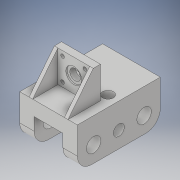
# Autodesk Inventor part: Y_Slider_Part_mit_Schrittmotor
Saved by Autodesk Inventor 2019 (Build 230136000, 136)
## iProperties
Created: 2018-08-19
Part Number: Y_Slider_Part_mit_Schrittmotor
Material: Generic
Document SubType Name: Modeling
Designer: Julia
Density: 1 g/cm^3
Appearance: Default
Author: Julia
Autodesk Inventor part; units mm, degrees
ref_plane "YZ Plane" through (0, 0, 0) normal (1, 0, 0) x (0, 1, 0)
ref_plane "XZ Plane" through (0, 0, 0) normal (0, 1, 0) x (-1, 0, 0)
ref_plane "XY Plane" through (0, 0, 0) normal (0, 0, 1) x (1, 0, 0)
sketch "Sketch1" plane through (0, 0, 0) normal (0, 1, 0) x (-1, 0, 0)
  line L0 (40, 57.5) -> (-40, 57.5)
  line L1 (-40, 57.5) -> (-40, -57.5)
  line L2 (-40, -57.5) -> (40, -57.5)
  line L3 (40, -57.5) -> (40, 57.5)
  point P0 (0, 0)
  point P1 (40, 0)
  point P2 (0, 57.5)
  dimension "d0" = 115
  dimension "d1" = 80
  constraints: 8 end point, 2 midpoint, 2 parallel, 1 horizontal, 1 horizontal alignment, 1 perpendicular, 1 vertical alignment
  measures "d0" distance of L2.end L0.start
  measures "d1" distance of L1.end L2.end
extrude "Extrusion1" add sketch "Sketch1" along normal blind 20
sketch "Sketch12" plane through (0, 0, 0) normal (0, -1, 0) x (1, 0, 0)
  line L0 (-40, 57.5) -> (-20, 57.5)
  line L1 (-20, 57.5) -> (-20, -57.5)
  line L2 (-20, -57.5) -> (-40, -57.5)
  line L3 (-40, -57.5) -> (-40, 57.5)
  line L4 (-40, -57.5) -> (-40, 57.5) projected
  line L5 (0, 100.8809) -> (0, -116.5773) construction
  line L6 (40, 57.5) -> (20, 57.5)
  line L7 (20, 57.5) -> (20, -57.5)
  line L8 (20, -57.5) -> (40, -57.5)
  line L9 (40, -57.5) -> (40, 57.5)
  point P0 (0, 0)
  point P1 (-40, 0)
  point P2 (0, 0)
  point P3 (-20, 0)
  dimension "d56" = 20
  dimension "d57" = 115
  constraints: 18 end point, 4 symmetric about line, 2 horizontal alignment, 2 midpoint, 2 parallel, 2 vertical, 1 collinear, 1 horizontal, 1 perpendicular
  measures "d56" distance of L0.start L0.end
  measures "d57" distance between parallel lines of L2 L0
extrude "Extrusion11" add sketch "Sketch12" along normal blind 37.5
sketch "Sketch13" plane through (-40, 0, 57.5) normal (-1, 0, 0) x (0, 0, 1)
  line L0 (0, 0) -> (-115, 0) projected
  point P0 (-57.5, 0)
  point P1 (-22.5, -15)
  point P2 (-92.5, -15)
  point P3 (-57.5, -15)
  point P4 (-57.5, 0)
  dimension "d129" = 35
  dimension "d130" = 35
  dimension "d131" = 15
  constraints: 2 horizontal alignment, 1 midpoint, 1 vertical alignment
  measures "d129" horizontal distance of point (-57.5, 0) point (-92.5, -15)
  measures "d130" horizontal distance of point (-22.5, -15) point (-57.5, 0)
  measures "d131" distance of point (-57.5, 0) point (-57.5, -15)
hole "Hole2" at (-40, -15, 35) at (-40, -15, -35) direction (1, 0, 0) diameter 20 end through all
hole "Hole3" at (-40, -15, 0) direction (1, 0, 0) diameter 15 end through all
sketch "Sketch19" plane through (0, 20, 0) normal (0, 1, 0) x (1, 0, 0)
  point P0 (0, 0)
  point P1 (25, 0)
  point P2 (-25, 0)
  dimension "d111" = 25
  dimension "d112" = 25
  constraints: 2 horizontal alignment
  measures "d111" distance of point (0, 0) point (25, 0)
  measures "d112" distance of point (-25, 0) point (0, 0)
hole "Hole6" at (25, 20, 0) at (-25, 20, 0) direction (0, -1, 0) diameter 15 depth 15
fillet "Fillet19" radius 20 4 edges at (-30, -37.5, -57.5) (30, -37.5, -57.5) (30, -37.5, 57.5) (-30, -37.5, 57.5)
sketch "Sketch20" plane through (0, 20, 0) normal (0, 1, 0) x (1, 0, 0)
  line L0 (-27, -22.5) -> (27, -22.5)
  line L1 (27, -22.5) -> (27, -12.5)
  line L2 (27, -12.5) -> (-27, -12.5)
  line L3 (-27, -12.5) -> (-27, -22.5)
  line L4 (-40, 57.5) -> (-40, -57.5) projected
  line L5 (40, -57.5) -> (40, 57.5) projected
  line L6 (-40, -57.5) -> (40, -57.5) projected
  point P0 (0, 0)
  point P1 (0, -12.5)
  dimension "d122" = 10
  dimension "d151" = 45
  dimension "d152" = 54
  constraints: 8 end point, 2 parallel, 1 horizontal, 1 midpoint, 1 perpendicular, 1 vertical alignment
  measures "d122" distance between parallel lines of L0 L2
  measures "d151" distance between parallel lines of L6 L2
  measures "d152" distance between parallel lines of L1 L3
extrude "Extrusion15" add sketch "Sketch20" along normal blind 44
sketch "Sketch21" plane through (-40, 20, 22.5) normal (0, 0, 1) x (1, 0, 0)
  circle A0 centre (40, 22) radius 7.5
  line L0 (20, -20) -> (60, -20) projected
  line L1 (13, 44) -> (67, 44) projected
  circle A1 centre (40, 22) radius 11
  point P0 (40, -20)
  point P1 (40, -20)
  point P2 (0, -20)
  point P3 (80, -20)
  point P4 (24.5, 37.5)
  point P5 (24.5, 6.5)
  point P6 (55.5, 6.5)
  point P7 (55.5, 37.5)
  dimension "d128" = 15
  dimension "d132" = 22
  dimension "d134" = 15.5
  dimension "d135" = 15.5
  dimension "d138" = 360
  dimension "d147" = 22
  constraints: 2 centre point, 1 coincident, 1 midpoint, 1 vertical alignment, 5 other
  measures "d128" diameter of A0
  measures "d132" distance from line of A0.centre L1
  measures "d134" horizontal distance of A0.centre point (24.5, 37.5)
  measures "d135" horizontal distance of A0.centre point (24.5, 37.5)
  measures "d147" diameter of A1
extrude "Extrusion16" cut sketch "Sketch21" against normal blind 50 contours A0
hole "Hole7" at (-15.5, 57.5, 22.5) at (-15.5, 26.5, 22.5) at (15.5, 26.5, 22.5) at (15.5, 57.5, 22.5) direction (0, 0, -1) diameter 5 depth 15
extrude "Extrusion17" cut sketch "Sketch21" against normal blind 2
sketch "Sketch24" plane through (0, 20, 0) normal (0, 1, 0) x (1, 0, 0)
  line L0 (-27, -22.5) -> (-22, -22.5)
  line L1 (-22, -22.5) -> (-22, -57.5)
  line L2 (-22, -57.5) -> (-27, -57.5)
  line L3 (-27, -57.5) -> (-27, -22.5)
  line L4 (-27, -22.5) -> (-27, -12.5) projected
  line L5 (27, -22.5) -> (-27, -22.5) projected
  line L6 (-40, -57.5) -> (40, -57.5) projected
  line L7 (22, -22.5) -> (27, -22.5)
  line L8 (27, -22.5) -> (27, -57.5)
  line L9 (27, -57.5) -> (22, -57.5)
  line L10 (22, -57.5) -> (22, -22.5)
  line L11 (27, -12.5) -> (27, -22.5) projected
  point P0 (0, 0)
  dimension "d155" = 5
  dimension "d156" = 5
  constraints: 16 end point, 6 collinear, 4 parallel, 2 horizontal, 2 perpendicular
  measures "d155" distance of L1.end L2.end
  measures "d156" distance between parallel lines of L8 L10
extrude "Extrusion18" add sketch "Sketch24" along normal blind 44 contours L0 L1 L2 L3 | L5 L8 L6 L10
sketch "Sketch25" plane through (27, 20, 57.5) normal (1, 0, 0) x (0, 0, -1)
  line L0 (35, 44) -> (0, 0)
  line L1 (0, 44) -> (35, 44)
  line L2 (0, 44) -> (0, 0)
  line L3 (45, 0) -> (45, 44) projected
  point P0 (57.5, -20)
  dimension "d161" = 10
  constraints: 6 end point, 3 coincident, 1 horizontal alignment
  measures "d161" distance from line of L3 L0.start
extrude "Extrusion19" cut sketch "Sketch25" against normal blind 100
body "Solid1"
